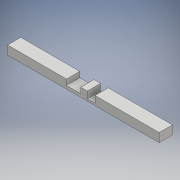
# Autodesk Inventor part: Cadru_4
Saved by Autodesk Inventor 2017 (Build 210142000, 142)
## iProperties
Created: 2017-06-13
Part Number: Cadru_4
Material: Generic
Document SubType Name: Modeling
Designer: crush
Density: 1 g/cm^3
Appearance: Default
Author: crush
Autodesk Inventor part; units mm, degrees
ref_plane "YZ Plane" through (0, 0, 0) normal (1, 0, 0) x (0, 1, 0)
ref_plane "XZ Plane" through (0, 0, 0) normal (0, 1, 0) x (-1, 0, 0)
ref_plane "XY Plane" through (0, 0, 0) normal (0, 0, 1) x (1, 0, 0)
sketch "Sketch1" plane through (0, 0, 0) normal (0, 1, 0) x (-1, 0, 0)
  line L0 (0, 0) -> (-690, 0)
  line L1 (-690, 0) -> (-690, -40)
  line L2 (-690, -40) -> (0, -40)
  line L3 (0, -40) -> (0, 0)
  dimension "d0" = 690
  dimension "d1" = 40
  constraints: 8 end point, 2 parallel, 1 horizontal, 1 perpendicular
  measures "d0" distance of L1.end L2.end
  measures "d1" distance of L2.end L0.start
extrude "Extrusion1" add sketch "Sketch1" along normal blind 60
sketch "Sketch3" plane through (0, 60, 0) normal (0, 1, 0) x (1, 0, 0)
  circle A0 centre (380.6828, 16.7692) radius 7.5
  line L0 (368.0221, 25.8207) -> (368.0221, 1.9407)
  line L1 (393.2421, 25.8207) -> (368.0221, 25.8207)
  line L2 (393.2421, 1.9407) -> (393.2421, 25.8207)
  line L3 (368.0221, 1.9407) -> (393.2421, 1.9407)
  line L4 (0, 0) -> (690, 0)
  line L5 (690, 40) -> (0, 40)
  line L6 (0, 40) -> (0, 0)
  line L7 (368.0221, 1.9407) -> (363.0221, 1.9407)
  line L8 (368.0221, 25.8207) -> (368.0221, 30.8207)
  line L9 (393.2421, 1.9407) -> (398.2421, 1.9407)
  line L10 (363.0221, 1.9407) -> (363.0221, 0)
  line L11 (398.2421, 1.9407) -> (398.2421, 0)
  line L12 (363.0221, 0) -> (398.2421, 0)
  line L13 (398.2421, 0) -> (398.2421, 30.8207)
  line L14 (398.2421, 30.8207) -> (363.0221, 30.8207)
  line L15 (363.0221, 30.8207) -> (363.0221, 0)
  point P0 (0, 40)
  dimension "d6" = 5
  dimension "d7" = 5
  dimension "d8" = 5
  constraints: 32 end point, 3 horizontal, 3 perpendicular, 2 parallel, 2 point on line, 1 centre point, 1 vertical
  measures "d6" distance of L0.end L7.end
  measures "d7" distance of L0.start L8.end
  measures "d8" distance of L2.start L9.end
extrude "Extrusion3" cut sketch "Sketch3" against normal blind 60 contours A0 | L1 L2 L3 L0 | L8 L14 L13 L9 L2 L1 | L0 L7 L15 L14 L8 | L3 L9 L11 L4 L10 L7
sketch "Sketch4" plane through (0, 0, 0) normal (0, -1, 0) x (1, 0, 0)
  line L0 (0, 0) -> (363.0221, 0) projected
  line L1 (333.0221, 0) -> (268.0221, 0)
  line L2 (268.0221, 0) -> (268.0221, -25)
  line L3 (268.0221, -25) -> (333.0221, -25)
  line L4 (333.0221, -25) -> (333.0221, 0)
  line L5 (363.0221, -30.8207) -> (363.0221, 0) projected
  dimension "d11" = 65
  dimension "d12" = 25
  dimension "d13" = 30
  constraints: 8 end point, 2 parallel, 1 horizontal, 1 perpendicular, 1 point on line
  measures "d11" distance of L2.end L3.end
  measures "d12" distance of L3.end L1.start
  measures "d13" distance between parallel lines of L5 L4
extrude "Extrusion4" cut sketch "Sketch4" against normal blind 60
body "Solid1"
